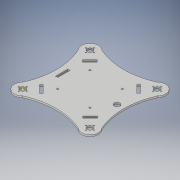
# Autodesk Inventor part: Base2
Saved by Autodesk Inventor 2019 (Build 230136000, 136)
## iProperties
Created: 2023-04-14
Part Number: Base2
Material: Generic
Document SubType Name: Modeling
Designer: Analuam
Density: 1 g/cm^3
Appearance: Default
Author: Analuam
Autodesk Inventor part; units mm, degrees
ref_plane "YZ Plane" through (0, 0, 0) normal (1, 0, 0) x (0, 1, 0)
ref_plane "XZ Plane" through (0, 0, 0) normal (0, 1, 0) x (-1, 0, 0)
ref_plane "XY Plane" through (0, 0, 0) normal (0, 0, 1) x (1, 0, 0)
sketch "Sketch1" plane through (0, 0, 0) normal (0, 1, 0) x (-1, 0, 0)
  arc A0 (-10.6066, -130.6066) -> (10.6066, -109.3934) centre (0, -120) ccw
  arc A1 (10.6066, -10.6066) -> (-10.6066, 10.6066) centre (0, 0) ccw
  arc A2 (-130.6066, -109.3934) -> (-109.3934, -130.6066) centre (-120, -120) ccw
  arc A3 (-109.3934, 10.6066) -> (-130.6066, -10.6066) centre (-120, 0) ccw
  arc A4 (10.6066, -10.6066) -> (10.6066, -109.3934) centre (120.3122, -60) ccw
  arc A5 (-10.6066, -130.6066) -> (-109.3934, -130.6066) centre (-60, -240.3122) ccw
  arc A6 (-109.3934, 10.6066) -> (-10.6066, 10.6066) centre (-60, 120.3122) ccw
  arc A7 (-130.6066, -109.3934) -> (-130.6066, -10.6066) centre (-244.217, -60) ccw
  circle A8 centre (7.1, 0) radius 1
  circle A9 centre (0, 7.1) radius 1
  circle A10 centre (-7.1, 0) radius 1
  circle A11 centre (0, -7.1) radius 1
  circle A12 centre (0, 0) radius 1.5
  circle A13 centre (-120, 0) radius 1.5
  circle A14 centre (-120, -120) radius 1.5
  circle A15 centre (0, -120) radius 1.5
  circle A16 centre (-120, 7.1) radius 1
  circle A17 centre (-127.1, 0) radius 1
  circle A18 centre (-120, -7.1) radius 1
  circle A19 centre (-112.9, 0) radius 1
  circle A20 centre (-127.1, -120) radius 1
  circle A21 centre (-120, -127.1) radius 1
  circle A22 centre (-112.9, -120) radius 1
  circle A23 centre (-120, -112.9) radius 1
  circle A24 centre (0, -127.1) radius 1
  circle A25 centre (7.1, -120) radius 1
  circle A26 centre (0, -112.9) radius 1
  circle A27 centre (-7.1, -120) radius 1
  line L0 (-21.7145, -8.1452) -> (-8.412, -21.4477)
  line L1 (-8.412, -21.4477) -> (-11.768, -24.8037)
  line L2 (-11.768, -24.8037) -> (-25.0705, -11.5012)
  line L3 (-25.0705, -11.5012) -> (-21.7145, -8.1452)
  line L4 (-95.1963, -11.768) -> (-108.4988, -25.0705)
  line L5 (-98.5523, -8.412) -> (-95.1963, -11.768)
  line L6 (-111.8548, -21.7145) -> (-98.5523, -8.412)
  line L7 (-108.4988, -25.0705) -> (-111.8548, -21.7145)
  line L8 (-108.232, -95.1963) -> (-94.9295, -108.4988)
  line L9 (-111.588, -98.5523) -> (-108.232, -95.1963)
  line L10 (-98.2855, -111.8548) -> (-111.588, -98.5523)
  line L11 (-94.9295, -108.4988) -> (-98.2855, -111.8548)
  line L12 (-24.8037, -108.232) -> (-11.5012, -94.9295)
  line L13 (-21.4477, -111.588) -> (-24.8037, -108.232)
  line L14 (-8.1452, -98.2855) -> (-21.4477, -111.588)
  line L15 (-11.5012, -94.9295) -> (-8.1452, -98.2855)
  circle A28 centre (-108.232, -60) radius 5
  line L16 (-9.5012, -49.1193) -> (-13.5012, -49.1193)
  line L17 (-13.5012, -49.1193) -> (-13.5012, -70.8807)
  line L18 (-13.5012, -70.8807) -> (-9.5012, -70.8807)
  line L19 (-9.5012, -70.8807) -> (-9.5012, -49.1193)
  line L20 (-9.5012, -49.1193) -> (-13.5012, -70.8807) construction
  line L21 (-13.5012, -49.1193) -> (-9.5012, -70.8807) construction
  circle A29 centre (-31.0935, -31.0935) radius 1.5
  circle A30 centre (-88.9065, -31.0935) radius 1.5
  circle A31 centre (-88.9065, -88.9065) radius 1.5
  circle A32 centre (-31.0935, -88.9065) radius 1.5
  point P0 (-60, -60)
  point P1 (-11.5012, -60)
  dimension "d13" = 360
  dimension "d19" = 360
  dimension "d23" = 360
  dimension "d29" = 360
  dimension "d31" = 10
  dimension "d32" = 4
  dimension "d33" = 3
  dimension "d36" = 360
  dimension "d48" = 57.813
  constraints: 44 end point, 33 centre point, 16 point on circle, 4 parallel, 2 coincident, 2 midpoint, 2 perpendicular, 1 horizontal, 93 other
  measures "d31" diameter of A28
  measures "d32" distance of L18.end L17.end
  measures "d33" diameter of A29
  measures "d48" distance of A32.centre A29.centre
extrude "Extrusion1" add sketch "Sketch1" along normal blind 3
sketch "Sketch2" plane through (0, 3, 0) normal (0, 1, 0) x (1, 0, 0)
  point P0 (0, 0)
sketch "Sketch3" plane through (0, 3, 0) normal (0, 1, 0) x (1, 0, 0)
  circle A0 centre (120, 120) radius 1.5 projected
  arc A1 (-10.6066, 10.6066) -> (10.6066, -10.6066) centre (0, 0) ccw projected
  line L0 (-10.6066, -10.6066) -> (130.6066, 130.6066)
  arc A2 (130.6066, 109.3934) -> (109.3934, 130.6066) centre (120, 120) ccw projected
  arc A3 (109.3934, -10.6066) -> (130.6066, 10.6066) centre (120, 0) ccw projected
  line L1 (130.6066, -10.6066) -> (-10.6066, 130.6066)
  circle A4 centre (0, 0) radius 5
  line L2 (60, 60) -> (63.3779, 59.6927)
  circle A5 centre (120, 0) radius 5
  circle A6 centre (120, 120) radius 5
  circle A7 centre (0, 120) radius 5
  dimension "d41" = 10
  dimension "d44" = 360
  constraints: 6 end point, 4 centre point, 3 point on circle, 1 coincident, 1 midpoint, 1 perpendicular, 9 other
  measures "d41" diameter of A4
sketch "Sketch4" plane through (0, 3, 0) normal (0, 1, 0) x (1, 0, 0)
  point P0 (0, 0)
extrude "Extrusion2" cut sketch "Sketch3" against normal blind 3 contours A0 L0 A6 | A0 L0 A6 | A5 L1 | L1 A5 | A4 L0 | L0 A4 | A7 L1 | L1 A7
body "Solid1"
